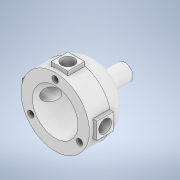
# Autodesk Inventor part: Large_mouse_poke
Saved by Autodesk Inventor 2020 (Build 240168000, 168)
## iProperties
Created: 2019-05-20
Part Number: Large_mouse_poke
Material: ABS Plastic
Document SubType Name: Modeling
Designer: Dammy
Density: 1.06 g/cm^3
Appearance: Smooth - White
Author: Dammy
Autodesk Inventor part; units mm, degrees
sketch "Sketch2" plane through (0, 0, 0) normal (0, 0, 1) x (1, 0, 0)
  circle A0 centre (0, 0) radius 13.5
  dimension "d0" = 27
  constraints: 1 centre point, 1 coincident
  measures "d0" diameter of A0
extrude "Base" add sketch "Sketch2" along normal blind 17.5
ref_plane "Work Plane1" through (13.5, 0, 0) normal (1, 0, 0) x (0, 1, 0)
sketch "Sketch3" plane through (13.5, 0, 0) normal (1, 0, 0) x (0, 1, 0)
  line L0 (13.5, 17.5) -> (-13.5, 17.5) projected
  line L1 (13.5, 0) -> (-13.5, 0) projected
  circle A0 centre (0, 12.5) radius 2.55
  point P0 (0, 0)
  dimension "d4" = 5.1
  dimension "d31" = 5
  constraints: 1 centre point
  measures "d4" diameter of A0
  measures "d31" distance from line of L0 A0.centre
extrude "IR hole" cut sketch "Sketch3" against normal through all
ref_plane "Work Plane2" through (0, 13.5, 0) normal (0, 1, 0) x (-1, 0, 0)
sketch "Sketch4" plane through (0, 13.5, 0) normal (0, 1, 0) x (-1, 0, 0)
  line L0 (13.5, 17.5) -> (-13.5, 17.5) construction
  line L1 (13.5, 0) -> (-13.5, 0) construction
  circle A0 centre (0, 12.5) radius 2.55
  point P0 (0, 0)
  dimension "d7" = 5.1
  dimension "d32" = 5
  constraints: 1 centre point
  measures "d7" diameter of A0
  measures "d32" distance from line of L0 A0.centre
extrude "LED Hole" cut sketch "Sketch4" against normal blind 13.5
sketch "Sketch7" plane through (0, 0, 0) normal (0, 0, -1) x (-1, 0, 0)
  circle A0 centre (0, 0) radius 1.25
  circle A1 centre (0, 0) radius 3.25
  dimension "d24" = 2.5
  dimension "d39" = 2
  constraints: 2 centre point, 2 coincident
  measures "d24" diameter of A0
  measures "d39" radial gap between concentric circles of A1 A0
extrude "Water Tube wall" add sketch "Sketch7" along normal blind 10
fillet "Fillet1" radius 9 1 edges at (-13.5, 0, 0)
ref_plane "Work Plane3" through (0, 0, 0) normal (0, 0, 1) x (1, 0, 0)
sketch "Sketch13" plane through (0, 0, 17.5) normal (0, 0, 1) x (1, 0, 0)
  circle A0 centre (0, 0) radius 1.25 projected
  circle A1 centre (0, 0) radius 9
  circle A2 centre (0, 0) radius 13.5 projected
  line L0 (-9, 0) -> (9, 0)
  point P0 (-1.25, 0)
  point P1 (1.25, 0)
  dimension "d40" = 4.5
  dimension "d66" = 18
  constraints: 2 end point, 2 point on circle, 1 centre point, 1 coincident, 1 horizontal
  measures "d40" radial gap between concentric circles of A2 A1
  measures "d66" diameter of A1
revolve "Inner cut out" cut sketch "Sketch13" angle 360 about axis through (-9, 0, 17.5) along (1, 0, 0) picked at (-6.3174, 0.8177) contours A0 L0 A1
sketch "Sketch14" plane through (0, 0, 17.5) normal (0, 0, 1) x (1, 0, 0)
  circle A0 centre (0, 11.1) radius 1.25
  line L0 (-18.9, 13.5) -> (18.9, 13.5) construction
  circle A1 centre (0, 0) radius 13.5 construction
  line L1 (0, 13.5) -> (0, 9) construction
  circle A2 centre (0, 0) radius 9 construction
  circle A3 centre (-9.6129, -5.55) radius 1.25
  circle A4 centre (9.6129, -5.55) radius 1.25
  circle A5 centre (0, 0) radius 11.1 construction
  dimension "d67" = 22.2
  dimension "d42" = 2.5
  dimension "d43" = 2.4
  dimension "d44" = 4.5
  dimension "d47" = 360
  constraints: 3 centre point, 2 end point, 2 vertical alignment, 1 coincident, 1 midpoint, 1 vertical, 12 other
  measures "d42" diameter of A0
  measures "d43" distance from line of L0 A0.centre
  measures "d44" distance of L1.start L1.end
extrude "Mount screw holes" cut sketch "Sketch14" against normal blind 5
ref_plane "Work Plane4" through (12.5, 0, 0) normal (1, 0, 0) x (0, 1, 0)
sketch "Sketch15" plane through (12.5, 0, 0) normal (1, 0, 0) x (0, 1, 0)
  circle A0 centre (0, 12.5) radius 2.55
  line L0 (13.5, 17.5) -> (-13.5, 17.5) projected
  line L1 (-3.3, 9.2) -> (3.3, 9.2)
  line L2 (3.3, 9.2) -> (3.3, 15.8)
  line L3 (3.3, 15.8) -> (-3.3, 15.8)
  line L4 (-3.3, 15.8) -> (-3.3, 9.2)
  line L5 (-3.3, 9.2) -> (3.3, 15.8) construction
  line L6 (3.3, 9.2) -> (-3.3, 15.8) construction
  point P0 (0, 0)
  dimension "d52" = 5
  dimension "d53" = 5.1
  dimension "d54" = 6.6
  dimension "d55" = 6.6
  constraints: 12 end point, 2 midpoint, 2 parallel, 1 centre point, 1 horizontal, 1 perpendicular
  measures "d52" distance from line of L0 A0.centre
  measures "d53" diameter of A0
  measures "d54" distance of L3.end L1.start
  measures "d55" distance of L2.end L3.end
extrude "Hole wall" add sketch "Sketch15" along normal blind 2.25
pattern_circular "Circular Pattern1" count 3 over 180 about axis through (0, 0, 0) along (0, 0, 1) of "Hole wall"
sketch "Sketch17" plane through (0, 0, 0) normal (0, 0, -1) x (-1, 0, 0)
  circle A0 centre (0, 0) radius 1.25 projected
  circle A1 centre (0, 0) radius 1.1
  dimension "d68" = 2.5
  constraints: 1 centre point, 1 coincident
  measures "d68" diameter of A0
extrude "Extrusion12" cut sketch "Sketch17" against normal blind 20 contours A0 | A1
equation "\"d8\" = 0.5 * d0"
equation "\"d52\" = d31"
equation "\"d53\" = d4"
equation "\"d55\" = d54"
body "Solid1"
